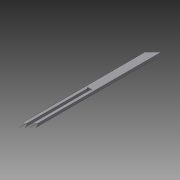
# Autodesk Inventor part: Effector_Arm_Ball
Saved by Autodesk Inventor 2014 (Build 180170000, 170)
## iProperties
Created: 2014-10-17
Part Number: Effector_Arm_Ball
Material: Generic
Document SubType Name: Modeling
Designer: ThatOtherGuy
Density: 1 g/cm^3
Appearance: Default
Author: ThatOtherGuy
Autodesk Inventor part; units mm, degrees
ref_plane "YZ Plane" through (0, 0, 0) normal (1, 0, 0) x (0, 1, 0)
ref_plane "XZ Plane" through (0, 0, 0) normal (0, 1, 0) x (-1, 0, 0)
ref_plane "XY Plane" through (0, 0, 0) normal (0, 0, 1) x (1, 0, 0)
sketch "Sketch1" plane through (0, 0, 0) normal (0, 0, 1) x (1, 0, 0)
  arc A0 (10, 0) -> (0, 0) centre (5, -3.3166) ccw
  arc A1 (0, 203.3668) -> (10, 203.3668) centre (5, 206.6834) ccw
  line L0 (0, 203.3668) -> (0, 0)
  line L1 (10, 0) -> (10, 203.3668)
  dimension "d0" = 10
  dimension "d1" = 6
  dimension "d2" = 210
  constraints: 4 end point, 4 point on circle, 2 centre point, 2 horizontal alignment, 2 vertical alignment, 1 equal radius, 1 parallel, 1 vertical
  measures "d0" distance between parallel lines of L0 L1
  measures "d1" radius of A0
  measures "d2" distance of A0.centre A1.centre
extrude "Extrusion1" add sketch "Sketch1" along normal blind 3.175
sketch "Sketch2" plane through (0, 0, 3.175) normal (0, 0, 1) x (1, 0, 0)
  arc A0 (10, 0) -> (0, 0) centre (5, -3.3166) ccw projected
  arc A1 (0, 203.3668) -> (10, 203.3668) centre (5, 206.6834) ccw projected
  line L0 (0, 203.3668) -> (0, 0) projected
  line L1 (2.4125, 2.0968) -> (2.4125, 2.6834)
  line L2 (2.4125, 2.6834) -> (3.4125, 2.6834)
  line L3 (3.4125, 2.6834) -> (3.4125, 100.0959)
  line L4 (3.4125, 101.6834) -> (6.5875, 101.6834)
  line L5 (6.5875, 100.0959) -> (6.5875, 2.6834)
  line L6 (6.5875, 2.6834) -> (7.5875, 2.6834)
  line L7 (7.5875, 2.6834) -> (7.5875, 2.0968)
  arc A2 (3.4125, 101.6834) -> (3.4125, 100.0959) centre (3.4125, 100.8896) ccw
  arc A3 (6.5875, 100.0959) -> (6.5875, 101.6834) centre (6.5875, 100.8896) ccw
  line L8 (10, 0) -> (10, 203.3668) projected
  line L9 (2.4125, 201.27) -> (2.4125, 200.6834)
  line L10 (2.4125, 200.6834) -> (7.5875, 200.6834)
  line L11 (7.5875, 200.6834) -> (7.5875, 201.27)
  point P0 (5, 101.6834)
  dimension "d6" = 3.175
  dimension "d7" = 1
  dimension "d8" = 210
  dimension "d9" = 105
  dimension "d10" = 0.7937
  constraints: 20 end point, 8 point on circle, 7 parallel, 6 collinear, 3 tangent, 2 centre point, 2 line through centre, 2 perpendicular, 1 equal radius, 1 midpoint, 1 vertical alignment
  measures "d6" distance between parallel lines of L5 L3
  measures "d7" distance between parallel lines of L3 L1
  measures "d8" distance of A1.centre A0.centre
  measures "d9" distance from line of A0.centre L4
  measures "d10" radius of A2
extrude "Extrusion2" cut sketch "Sketch2" against normal up to next contours A0 L1 L2 L3 A2 L4 A3 L5 L6 L7 | L11 L10 A1 | L10 L9 A1
fillet "Fillet1" radius 0.7937 4 edges at (2.4125, 2.6834, 1.5875) (7.5875, 2.6834, 1.5875) (2.4125, 200.6834, 1.5875) (7.5875, 200.6834, 1.5875)
fillet "Fillet1" radius 0.5 4 edges at (0, 0, 1.5875) (10, 0, 1.5875) (10, 203.3668, 1.5875) (0, 203.3668, 1.5875)
equation "\"d3\" = THICKA"
equation "\"d6\" = THICKA"
equation "\"d9\" = 0.5 * d8"
equation "\"d11\" = THICKA"
equation "\"THICKA\" = 3.175"
equation "\"THICKB\" = 6.731"
equation "\"THICKC\" = 12.7"
equation "\"MAGDIA\" = 9.5"
equation "\"BALLDIA\" = 12"
body "Solid1"
